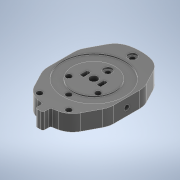
# Autodesk Inventor part: Platform
Saved by Autodesk Inventor 2022 (Build 260153000, 153)
## iProperties
Created: 2022-03-02
Part Number: Platform
Material: Genérico
Document SubType Name: Modeling
Designer: JK
Density: 1 g/cm^3
Appearance: Suave - Negro
Author: JK
Autodesk Inventor part; units mm, degrees
ref_plane "YZ Plane" through (0, 0, 0) normal (1, 0, 0) x (0, 1, 0)
ref_plane "XZ Plane" through (0, 0, 0) normal (0, 1, 0) x (-1, 0, 0)
ref_plane "XY Plane" through (0, 0, 0) normal (0, 0, 1) x (1, 0, 0)
sketch "Boceto1" plane through (0, 0, 0) normal (0, 1, 0) x (-1, 0, 0)
  circle A0 centre (0, 0) radius 19.876
  circle A1 centre (0, 0) radius 32.85
  circle A2 centre (0, 0) radius 50
  dimension "d0" = 65.7
  dimension "d1" = 100
  constraints: 3 centre point, 3 coincident
  measures "d0" diameter of A1
  measures "d1" diameter of A2
extrude "Extrusión1" add sketch "Boceto1" along normal blind 17 contours A0 | A1 | A2
sketch "Boceto2" plane through (0, 17, 0) normal (0, 1, 0) x (1, 0, 0)
  circle A0 centre (0, 0) radius 32.875
  circle A1 centre (0, 0) radius 22.45
  dimension "d4" = 65.75
  dimension "d5" = 44.9
  constraints: 2 centre point, 2 coincident
  measures "d4" diameter of A0
  measures "d5" diameter of A1
extrude "Extrusión2" cut sketch "Boceto2" against normal blind 1.4
sketch "Boceto3" plane through (0, 17, 0) normal (0, 1, 0) x (1, 0, 0)
  circle A0 centre (0, 0) radius 22.45 projected
extrude "Extrusión3" add sketch "Boceto3" along normal blind 1
sketch "Boceto4" plane through (0, 18, 0) normal (0, 1, 0) x (1, 0, 0)
  circle A0 centre (0, 0) radius 4
  line L0 (2.9, -2.755) -> (2.9, 2.755)
  dimension "d11" = 8
  dimension "d12" = 2.9
  constraints: 2 end point, 2 point on circle, 1 centre point, 1 coincident, 1 vertical
  measures "d11" diameter of A0
  measures "d12" distance from line of point (0, 0) L0
extrude "Extrusión4" cut sketch "Boceto4" against normal through all contours L0 A0 picked at (-0.156, 0.667)
sketch "Boceto5" plane through (0, 18, 0) normal (0, 1, 0) x (1, 0, 0)
  arc A0 (2.9, 2.755) -> (2.9, -2.755) centre (0, 0) ccw projected
  line L0 (2.9, 2.755) -> (2.9, -2.755) projected
  arc A1 (3, 2.7946) -> (3, -2.7946) centre (0, 0) ccw
  line L1 (3, 2.7946) -> (3, -2.7946)
  dimension "d15" = 0.1
  constraints: 2 end point, 2 point on circle, 1 centre point, 1 other
  measures "d15" radial gap between concentric circles of A1 A0
extrude "Extrusión5" cut sketch "Boceto5" against normal through all contours L0 A0 | L1 A1
sketch "Boceto6" plane through (0, 0, 0) normal (0, -1, 0) x (1, 0, 0)
  line L0 (-35, 64.067) -> (35, 64.067)
  line L1 (35, 64.067) -> (35, -64.067)
  line L2 (35, -64.067) -> (-35, -64.067)
  line L3 (-35, -64.067) -> (-35, 64.067)
  line L4 (-35, 64.067) -> (35, -64.067) construction
  line L5 (35, 64.067) -> (-35, -64.067) construction
  arc A0 (3, 2.7946) -> (3, -2.7946) centre (0, 0) ccw projected
  line L6 (3, 2.7946) -> (3, -2.7946) projected
  circle A1 centre (0, 0) radius 50 projected
  point P0 (0, 0)
  point P1 (-35, 35.7071)
  point P2 (-35, -35.7071)
  point P3 (35, 35.7071)
  point P4 (35, -35.7071)
  dimension "d19" = 70
  constraints: 12 end point, 3 midpoint, 2 parallel, 1 coincident, 1 horizontal, 1 perpendicular
  measures "d19" distance of L1.end L2.end
extrude "Extrusión6" cut sketch "Boceto6" against normal through all contours L3 A1 | A1 L1
chamfer "Chaflán1" distance 17 angle 45 4 edges at (-35, 8.5, 35.7071) (-35, 8.5, -35.7071) (35, 8.5, -35.7071) (35, 8.5, 35.7071)
fillet "Empalme2" radius 20 8 edges at (-21.0133, 8.5, 45.3701) (-35, 8.5, 18.7071) (-35, 8.5, -18.7071) (-21.0133, 8.5, -45.3701) (21.0133, 8.5, -45.3701) (35, 8.5, -18.7071) (35, 8.5, 18.7071) (21.0133, 8.5, 45.3701)
sketch "Boceto8" plane through (0, 18, 0) normal (0, 1, 0) x (1, 0, 0)
  arc A0 (3, 2.7946) -> (3, -2.7946) centre (0, 0) ccw projected
  line L0 (3, 2.7946) -> (3, -2.7946) projected
sketch "Boceto9" plane through (0, 17, 0) normal (0, 1, 0) x (1, 0, 0)
  circle A0 centre (0, 41) radius 2.7
  circle A1 centre (0, 15) radius 2.7
  circle A2 centre (0, -15) radius 2.7
  point P0 (0, 0)
  dimension "d30" = 5.4
  dimension "d31" = 5.4
  dimension "d32" = 15
  dimension "d33" = 26
  dimension "d45" = 15
  constraints: 3 centre point, 1 equal radius
  measures "d30" diameter of A0
  measures "d31" diameter of A1
  measures "d32" distance of A1.centre point (0, 0)
  measures "d33" distance of A1.centre A0.centre
  measures "d45" distance of A2.centre point (0, 0)
extrude "Extrusión8" cut sketch "Boceto9" along normal blind 15 and the other way blind 27.75
sketch "Boceto13" plane through (0, 17, 0) normal (0, 1, 0) x (1, 0, 0)
  circle A0 centre (0, 41) radius 2.7 projected
  circle A1 centre (0, 41) radius 4.6
  circle A2 centre (0, 15) radius 2.7 projected
  circle A3 centre (0, 15) radius 4.6
  circle A4 centre (0, -15) radius 2.7 projected
  circle A5 centre (0, -15) radius 4.6
  point P0 (0, 0)
  dimension "d38" = 9.2
  dimension "d39" = 9.2
  constraints: 3 centre point, 3 coincident, 1 equal radius
  measures "d38" diameter of A1
  measures "d39" diameter of A3
extrude "Extrusión9" cut sketch "Boceto13" along normal blind 2 and the other way blind 2 contours A0 | A1 | A3 | A4 | A5
sketch "Boceto14" plane through (0, 18, 0) normal (0, 1, 0) x (1, 0, 0)
  circle A0 centre (0, 0) radius 9
  dimension "d46" = 18
  constraints: 1 centre point, 1 coincident
  measures "d46" diameter of A0
extrude "Extrusión10" add sketch "Boceto14" along normal blind 2.5
sketch "Boceto15" plane through (0, 0, 0) normal (0, -1, 0) x (1, 0, 0)
  line L0 (3, -2.7946) -> (3, 2.7946) projected
  arc A0 (3, 2.7946) -> (3, -2.7946) centre (0, 0) ccw projected
extrude "Extrusión11" cut sketch "Boceto15" against normal through all
fillet "Empalme3" radius 2 1 edges at (-9, 18, 0)
sketch "Boceto16" plane through (0, 20.5, 0) normal (0, 1, 0) x (1, 0, 0)
  circle A0 centre (0, 0) radius 4.15
  constraints: 1 centre point, 1 coincident
extrude "Extrusión12" cut sketch "Boceto16" against normal blind 2
sketch "Boceto17" plane through (0, 18, 0) normal (0, 1, 0) x (1, 0, 0)
  arc A0 (1.9376, -10.828) -> (1.9376, 10.828) centre (0, 0) ccw projected
  arc A1 (-1.9376, -10.828) -> (1.9376, -10.828) centre (0, -15) ccw projected
  arc A2 (-1.9376, 10.828) -> (-1.9376, -10.828) centre (0, 0) ccw projected
  arc A3 (1.9376, 10.828) -> (-1.9376, 10.828) centre (0, 15) ccw projected
  circle A4 centre (0, 0) radius 22.45 projected
extrude "Extrusión13" cut sketch "Boceto17" against normal up to surface (1 mm away)
sketch "Boceto18" plane through (0, 17, 0) normal (0, 1, 0) x (1, 0, 0)
  circle A0 centre (0, 0) radius 13.4678
  constraints: 1 centre point, 1 coincident
extrude "Extrusión14" cut sketch "Boceto18" along normal blind 17.5
sketch "Boceto19" plane through (0, 17, 0) normal (0, 1, 0) x (1, 0, 0)
  circle A0 centre (0, 0) radius 4.1
  arc A1 (3, 2.7946) -> (3, -2.7946) centre (0, 0) ccw projected
  constraints: 1 centre point, 1 coincident, 1 concentric
extrude "Extrusión15" cut sketch "Boceto19" against normal blind 3
sketch "Boceto20" plane through (0, 17, 0) normal (0, 1, 0) x (1, 0, 0)
  circle A0 centre (-15.5, -42) radius 1.7
  point P0 (0, 0)
  point P1 (0, -26.5)
  dimension "d60" = 15.5
  dimension "d61" = 15.5
  dimension "d62" = 3.4
  dimension "d84" = 42
  constraints: 1 centre point, 1 vertical alignment
  measures "d60" horizontal distance of A0.centre point (0, -26.5)
  measures "d61" horizontal distance of A0.centre point (0, -26.5)
  measures "d62" diameter of A0
  measures "d84" vertical distance of A0.centre point (0, 0)
extrude "Extrusión16" cut sketch "Boceto20" against normal through all
sketch "Boceto21" plane through (0, 17, 0) normal (0, 1, 0) x (1, 0, 0)
  line L0 (11.1, 4.05) -> (6.9, 4.05)
  line L1 (6.9, 4.05) -> (6.9, -4.05)
  line L2 (6.9, -4.05) -> (11.1, -4.05)
  line L3 (11.1, -4.05) -> (11.1, 4.05)
  line L4 (11.1, 4.05) -> (6.9, -4.05) construction
  line L5 (6.9, 4.05) -> (11.1, -4.05) construction
  point P0 (0, 0)
  point P1 (9, 0)
  dimension "d65" = 8.1
  dimension "d66" = 4.2
  dimension "d107" = 9
  constraints: 12 end point, 2 midpoint, 2 parallel, 1 horizontal, 1 perpendicular
  measures "d65" distance between parallel lines of L2 L0
  measures "d66" distance between parallel lines of L3 L1
  measures "d107" distance of point (0, 0) point (9, 0)
extrude "Extrusión17" cut sketch "Boceto21" against normal blind 14
sketch "Boceto22" plane through (35, 0, 13.7798) normal (1, 0, 0) x (0, 0, -1)
  circle A0 centre (13.7798, 7.6) radius 2.7
  line L0 (17.8298, 3) -> (9.7298, 3) projected
  point P0 (13.7798, 0)
  point P1 (13.7798, 3)
  dimension "d69" = 5.4
  dimension "d70" = 4.6
  constraints: 1 centre point, 1 midpoint, 1 vertical alignment
  measures "d69" diameter of A0
  measures "d70" distance from line of L0 A0.centre
extrude "Extrusión18" cut sketch "Boceto22" against normal blind 35.25
sketch "Boceto23" plane through (0, 17, 0) normal (0, 1, 0) x (1, 0, 0)
  circle A0 centre (0, -26.5) radius 3
  circle A1 centre (-15.5, -42) radius 1.7 projected
  point P0 (0, 0)
  dimension "d73" = 15.5
  dimension "d74" = 15.5
  dimension "d81" = 6
  constraints: 1 centre point
  measures "d73" horizontal distance of A1.centre A0.centre
  measures "d74" horizontal distance of A1.centre A0.centre
  measures "d81" diameter of A0
extrude "Extrusión20" cut sketch "Boceto23" against normal through all contours A0
sketch "Boceto24" plane through (0, 17, 0) normal (0, 1, 0) x (1, 0, 0)
  circle A0 centre (-15.5, -42) radius 1.7 projected
  circle A1 centre (-15.5, -42) radius 3
  point P0 (0, 0)
  dimension "d78" = 6
  constraints: 1 centre point, 1 coincident
  measures "d78" diameter of A1
extrude "Extrusión19" cut sketch "Boceto24" against normal blind 4
pattern_circular "Patrón circular1" count 4 over 360 about axis through (0, 17, 26.5) along (0, 1, 0) of "Extrusión16", "Extrusión20", "Extrusión19"
sketch "Boceto33" plane through (0, 0, 0) normal (0, -1, 0) x (1, 0, 0)
  circle A0 centre (0, 26.5) radius 3 projected
  circle A1 centre (0, 26.5) radius 8
  point P0 (0, 0)
  dimension "d114" = 16
  constraints: 1 centre point, 1 coincident
  measures "d114" diameter of A1
extrude "Extrusión28" cut sketch "Boceto33" against normal blind 10 contours A0 | A1
sketch "Boceto34" plane through (0, 0, 0) normal (0, -1, 0) x (1, 0, 0)
  circle A0 centre (0, 15) radius 2.7 projected
  point P0 (0, 0)
extrude "Extrusión29" add sketch "Boceto34" against normal up to surface (17 mm away)
sketch "Boceto35" plane through (0, 17, 0) normal (0, 1, 0) x (1, 0, 0)
  circle A0 centre (0, -15) radius 4.6 projected
  point P0 (0, 0)
extrude "Extrusión30" add sketch "Boceto35" against normal blind 3.75
pattern_circular "Patrón circular2" count 2 over 360 about axis through (0, 18, 0) along (0, -1, 0) of "Extrusión17", "Extrusión18"
sketch "Boceto36" plane through (0, 0, 0) normal (0, -1, 0) x (1, 0, 0)
  arc A0 (11.5251, 48.6536) -> (-11.5251, 48.6536) centre (0, 0) ccw projected
  line L0 (-4, 42) -> (4, 42)
  line L1 (4, 42) -> (4, 58)
  line L2 (4, 58) -> (-4, 58)
  line L3 (-4, 58) -> (-4, 42)
  line L4 (-4, 42) -> (4, 58) construction
  line L5 (4, 42) -> (-4, 58) construction
  point P0 (-4, 49.8397)
  point P1 (4, 49.8397)
  point P2 (0, 50)
  dimension "d125" = 8
  dimension "d129" = 8
  constraints: 12 end point, 2 parallel, 1 horizontal, 1 midpoint, 1 perpendicular, 1 point on circle
  measures "d125" distance of L1.end L2.end
  measures "d129" distance from line of L2 point (0, 50)
extrude "Extrusión31" add sketch "Boceto36" against normal up to surface (17 mm away) contours A0 L3 L2 L1
fillet "Empalme5" radius 2 4 edges at (-4, 8.5, 58) (4, 8.5, 58) (-4, 8.5, 49.8397) (4, 8.5, 49.8397)
sketch "Boceto37" plane through (0, 0, 0) normal (0, -1, 0) x (1, 0, 0)
  arc A0 (3, 2.7946) -> (3, -2.7946) centre (0, 0) ccw projected
  circle A1 centre (0, 0) radius 4.1
  point P0 (3, -2.7946)
  constraints: 1 centre point, 1 coincident, 1 concentric
extrude "Extrusión32" cut sketch "Boceto37" against normal through all
sketch "Boceto30" plane through (0, 17, 0) normal (0, 1, 0) x (1, 0, 0)
  circle A0 centre (0, 0) radius 6.9
  constraints: 1 centre point, 1 coincident
sketch "Boceto31" plane through (0, 17, 0) normal (0, 1, 0) x (1, 0, 0)
  circle A0 centre (0, 0) radius 6.9 projected
  circle A1 centre (0, 0) radius 4.1 projected
sketch "Boceto32" plane through (0, 14, 0) normal (0, 1, 0) x (0, 0, -1)
  line L0 (-2.7946, -3) -> (2.7946, -3) projected
  arc A0 (-2.7946, -3) -> (2.7946, -3) centre (0, 0) ccw projected
sketch "Boceto26" plane through (0, 17, 0) normal (0, 1, 0) x (1, 0, 0)
  line L0 (24, -87.6765) -> (-24, -87.6765)
  line L1 (-24, -87.6765) -> (-24, -39.6765)
  line L2 (-24, -39.6765) -> (24, -39.6765)
  line L3 (24, -39.6765) -> (24, -87.6765)
  line L4 (24, -87.6765) -> (-24, -39.6765) construction
  line L5 (-24, -87.6765) -> (24, -39.6765) construction
  line L6 (32.7111, -23.0706) -> (24.6261, -38.4829) projected
  point P0 (0, 0)
  point P1 (0, -63.6765)
  point P2 (0, -63.6765)
  dimension "d85" = 48
  dimension "d86" = 48
  constraints: 12 end point, 3 midpoint, 2 parallel, 1 horizontal, 1 perpendicular, 1 point on line, 1 vertical alignment
  measures "d85" distance of L1.end L2.end
  measures "d86" distance of L0.end L1.end
sketch "Boceto27" plane through (0, 17, 0) normal (0, 1, 0) x (1, 0, 0)
  circle A0 centre (0, -63.6765) radius 3
  line L0 (-19, -87.6765) -> (19, -87.6765) projected
  circle A1 centre (-15.5, -79.4365) radius 1.7
  circle A2 centre (-15.5, -48.4365) radius 1.7
  circle A3 centre (15.5, -79.4365) radius 1.7
  circle A4 centre (15.5, -48.4365) radius 1.7
  point P0 (0, 0)
  dimension "d90" = 6
  dimension "d91" = 24
  dimension "d92" = 3.4
  dimension "d93" = 15.5
  dimension "d94" = 31
  dimension "d95" = 15.5
  constraints: 5 centre point, 3 equal radius, 2 horizontal alignment, 2 vertical alignment
  measures "d90" diameter of A0
  measures "d91" distance from line of L0 A0.centre
  measures "d92" diameter of A1
  measures "d93" horizontal distance of A1.centre A0.centre
  measures "d94" distance of A2.centre A1.centre
  measures "d95" horizontal distance of A3.centre A0.centre
sketch "Boceto28" plane through (0, 17, 0) normal (0, 1, 0) x (1, 0, 0)
  line L0 (-13.8, -83.4365) -> (-17.2, -83.4365)
  line L1 (-17.2, -83.4365) -> (-17.2, -75.4365)
  line L2 (-17.2, -75.4365) -> (-13.8, -75.4365)
  line L3 (-13.8, -75.4365) -> (-13.8, -83.4365)
  circle A0 centre (-15.5, -79.4365) radius 1.7 projected
  line L4 (-13.8, -83.4365) -> (-17.2, -75.4365) construction
  line L5 (-17.2, -83.4365) -> (-13.8, -75.4365) construction
  line L6 (-13.8, -52.4365) -> (-17.2, -52.4365)
  line L7 (-17.2, -52.4365) -> (-17.2, -44.4365)
  line L8 (-17.2, -44.4365) -> (-13.8, -44.4365)
  line L9 (-13.8, -44.4365) -> (-13.8, -52.4365)
  circle A1 centre (-15.5, -48.4365) radius 1.7 projected
  line L10 (-13.8, -52.4365) -> (-17.2, -44.4365) construction
  line L11 (-17.2, -52.4365) -> (-13.8, -44.4365) construction
  line L12 (3, -67.6765) -> (-3, -67.6765)
  line L13 (-3, -67.6765) -> (-3, -59.6765)
  line L14 (-3, -59.6765) -> (3, -59.6765)
  line L15 (3, -59.6765) -> (3, -67.6765)
  circle A2 centre (0, -63.6765) radius 3 projected
  line L16 (3, -67.6765) -> (-3, -59.6765) construction
  line L17 (-3, -67.6765) -> (3, -59.6765) construction
  line L18 (17.2, -52.4365) -> (13.8, -52.4365)
  line L19 (13.8, -52.4365) -> (13.8, -44.4365)
  line L20 (13.8, -44.4365) -> (17.2, -44.4365)
  line L21 (17.2, -44.4365) -> (17.2, -52.4365)
  circle A3 centre (15.5, -48.4365) radius 1.7 projected
  line L22 (17.2, -52.4365) -> (13.8, -44.4365) construction
  line L23 (13.8, -52.4365) -> (17.2, -44.4365) construction
  line L24 (17.2, -83.4365) -> (13.8, -83.4365)
  line L25 (13.8, -83.4365) -> (13.8, -75.4365)
  line L26 (13.8, -75.4365) -> (17.2, -75.4365)
  line L27 (17.2, -75.4365) -> (17.2, -83.4365)
  circle A4 centre (15.5, -79.4365) radius 1.7 projected
  line L28 (17.2, -83.4365) -> (13.8, -75.4365) construction
  line L29 (13.8, -83.4365) -> (17.2, -75.4365) construction
  circle A5 centre (-15.5, -83.4365) radius 1.7
  circle A6 centre (-15.5, -75.4365) radius 1.7
  circle A7 centre (-15.5, -52.4365) radius 1.7
  circle A8 centre (-15.5, -44.4365) radius 1.7
  circle A9 centre (15.5, -52.4365) radius 1.7
  circle A10 centre (15.5, -44.4365) radius 1.7
  circle A11 centre (15.5, -83.4365) radius 1.7
  circle A12 centre (15.5, -75.4365) radius 1.7
  circle A13 centre (-15.5, -79.4365) radius 1.7 projected
  circle A14 centre (0, -67.6765) radius 3
  circle A15 centre (0, -59.6765) radius 3
  point P0 (0, 0)
  dimension "d98" = 8
  constraints: 60 end point, 20 midpoint, 10 parallel, 5 equal length, 5 horizontal, 5 perpendicular, 2 point on line, 2 tangent, 30 other
  measures "d98" distance of L0.end L1.end
sketch "Boceto29" plane through (0, 17, 0) normal (0, 1, 0) x (1, 0, 0)
  line L0 (17.2, -44.4365) -> (17.2, -52.4365) projected
  arc A0 (13.8, -52.4365) -> (17.2, -52.4365) centre (15.5, -52.4365) ccw projected
  line L1 (13.8, -52.4365) -> (13.8, -44.4365) projected
  arc A1 (17.2, -44.4365) -> (13.8, -44.4365) centre (15.5, -44.4365) ccw projected
  line L2 (13.8, -83.4365) -> (13.8, -75.4365) projected
  arc A2 (17.2, -75.4365) -> (13.8, -75.4365) centre (15.5, -75.4365) ccw projected
  line L3 (17.2, -75.4365) -> (17.2, -83.4365) projected
  arc A3 (13.8, -83.4365) -> (17.2, -83.4365) centre (15.5, -83.4365) ccw projected
  line L4 (3, -59.6765) -> (3, -67.6765) projected
  arc A4 (-3, -67.6765) -> (3, -67.6765) centre (0, -67.6765) ccw projected
  line L5 (-3, -67.6765) -> (-3, -59.6765) projected
  arc A5 (3, -59.6765) -> (-3, -59.6765) centre (0, -59.6765) ccw projected
  line L6 (-17.2, -83.4365) -> (-17.2, -75.4365) projected
  arc A6 (-13.8, -75.4365) -> (-17.2, -75.4365) centre (-15.5, -75.4365) ccw projected
  line L7 (-13.8, -75.4365) -> (-13.8, -83.4365) projected
  arc A7 (-17.2, -83.4365) -> (-13.8, -83.4365) centre (-15.5, -83.4365) ccw projected
  line L8 (-17.2, -52.4365) -> (-17.2, -44.4365) projected
  arc A8 (-13.8, -44.4365) -> (-17.2, -44.4365) centre (-15.5, -44.4365) ccw projected
  line L9 (-13.8, -44.4365) -> (-13.8, -52.4365) projected
  arc A9 (-17.2, -52.4365) -> (-13.8, -52.4365) centre (-15.5, -52.4365) ccw projected
  circle A10 centre (0, 0) radius 32.875 projected
  arc A11 (19, -87.6765) -> (24, -82.6765) centre (19, -82.6765) ccw projected
  line L10 (24, -82.6765) -> (24, -40.4042) projected
  arc A12 (24, -40.4042) -> (23.9468, -39.6765) centre (19, -40.4042) ccw projected
  arc A13 (23.9468, -39.6765) -> (24.6261, -38.4829) centre (6.915, -29.1922) ccw projected
  line L11 (32.7111, -23.0706) -> (24.6261, -38.4829) projected
  arc A14 (32.7111, -23.0706) -> (35, -13.7798) centre (15, -13.7798) ccw projected
  line L12 (35, -13.7798) -> (35, 13.7798) projected
  arc A15 (35, 13.7798) -> (32.7111, 23.0706) centre (15, 13.7798) ccw projected
  line L13 (24.6261, 38.4829) -> (32.7111, 23.0706) projected
  arc A16 (24.6261, 38.4829) -> (11.5251, 48.6536) centre (6.915, 29.1922) ccw projected
  arc A17 (11.5251, 48.6536) -> (-11.5251, 48.6536) centre (0, 0) ccw projected
  arc A18 (-11.5251, 48.6536) -> (-24.6261, 38.4829) centre (-6.915, 29.1922) ccw projected
  line L14 (-32.7111, 23.0706) -> (-24.6261, 38.4829) projected
  arc A19 (-32.7111, 23.0706) -> (-35, 13.7798) centre (-15, 13.7798) ccw projected
  line L15 (-35, 13.7798) -> (-35, -13.7798) projected
  arc A20 (-35, -13.7798) -> (-32.7111, -23.0706) centre (-15, -13.7798) ccw projected
  line L16 (-24.6261, -38.4829) -> (-32.7111, -23.0706) projected
  arc A21 (-24.6261, -38.4829) -> (-23.9468, -39.6765) centre (-6.915, -29.1922) ccw projected
  arc A22 (-23.9468, -39.6765) -> (-24, -40.4042) centre (-19, -40.4042) ccw projected
  line L17 (-24, -40.4042) -> (-24, -82.6765) projected
  arc A23 (-24, -82.6765) -> (-19, -87.6765) centre (-19, -82.6765) ccw projected
  line L18 (-19, -87.6765) -> (19, -87.6765) projected
  circle A24 centre (0, 41) radius 4.6 projected
  line L19 (-18.7, -75.4365) -> (-18.7, -83.4365)
  arc A25 (-18.7, -83.4365) -> (-12.3, -83.4365) centre (-15.5, -83.4365) ccw
  line L20 (-12.3, -83.4365) -> (-12.3, -75.4365)
  arc A26 (-12.3, -75.4365) -> (-18.7, -75.4365) centre (-15.5, -75.4365) ccw
  line L21 (-18.7, -44.4365) -> (-18.7, -52.4365)
  arc A27 (-18.7, -52.4365) -> (-12.3, -52.4365) centre (-15.5, -52.4365) ccw
  line L22 (-12.3, -52.4365) -> (-12.3, -44.4365)
  arc A28 (-12.3, -44.4365) -> (-18.7, -44.4365) centre (-15.5, -44.4365) ccw
  line L23 (12.3, -44.4365) -> (12.3, -52.4365)
  arc A29 (12.3, -52.4365) -> (18.7, -52.4365) centre (15.5, -52.4365) ccw
  line L24 (18.7, -52.4365) -> (18.7, -44.4365)
  arc A30 (18.7, -44.4365) -> (12.3, -44.4365) centre (15.5, -44.4365) ccw
  line L25 (12.3, -75.4365) -> (12.3, -83.4365)
  arc A31 (12.3, -83.4365) -> (18.7, -83.4365) centre (15.5, -83.4365) ccw
  line L26 (18.7, -83.4365) -> (18.7, -75.4365)
  arc A32 (18.7, -75.4365) -> (12.3, -75.4365) centre (15.5, -75.4365) ccw
  dimension "d101" = 1.5
  dimension "d102" = 1.5
  dimension "d103" = 1.5
  dimension "d104" = 1.5
  constraints: 1 centre point, 1 coincident
  measures "d101" distance between parallel lines of L6 L19
  measures "d102" distance between parallel lines of L8 L21
  measures "d103" distance between parallel lines of L25 L2
  measures "d104" distance between parallel lines of L23 L1
